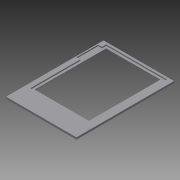
# Autodesk Inventor part: TouchBottom
Saved by Autodesk Inventor 2014 SP1 (Build 180222100, 222)
## iProperties
Created: 2014-03-24
Part Number: TouchBottom
Material: Generic
Document SubType Name: Modeling
Designer: patrigg
Density: 1 g/cm^3
Appearance: Default
Author: patrigg
Autodesk Inventor part; units mm, degrees
ref_plane "YZ Plane" through (0, 0, 0) normal (1, 0, 0) x (0, 1, 0)
ref_plane "XZ Plane" through (0, 0, 0) normal (0, 1, 0) x (-1, 0, 0)
ref_plane "XY Plane" through (0, 0, 0) normal (0, 0, 1) x (1, 0, 0)
sketch "Sketch1" plane through (0, 0, 0) normal (0, 1, 0) x (-1, 0, 0)
  line L0 (-32.5, -45) -> (32.5, -45)
  line L1 (32.5, -45) -> (32.5, 45)
  line L2 (32.5, 45) -> (-32.5, 45)
  line L3 (-32.5, 45) -> (-32.5, -45)
  line L4 (-32.5, -45) -> (32.5, 45) construction
  line L5 (32.5, -45) -> (-32.5, 45) construction
  point P0 (0, 0)
  dimension "d0" = 65
  dimension "d1" = 90
  constraints: 12 end point, 2 midpoint, 2 parallel, 1 horizontal, 1 perpendicular
  measures "d0" distance of L2.end L1.end
  measures "d1" distance of L1.end L0.end
extrude "Extrusion1" add sketch "Sketch1" along normal blind 1.8
sketch "Sketch2" plane through (0, 1.8, 0) normal (0, 1, 0) x (1, 0, 0)
  line L0 (32.5, 45) -> (-32.5, 45) projected
  line L1 (-28, -27) -> (28, -27)
  line L2 (28, -27) -> (28, 43)
  line L3 (28, 43) -> (-28, 43)
  line L4 (-28, 43) -> (-28, -27)
  line L5 (-28, -27) -> (28, 43) construction
  line L6 (28, -27) -> (-28, 43) construction
  line L7 (32.5, -45) -> (32.5, 45) projected
  point P0 (0, 0)
  point P1 (0, 8)
  point P2 (0, 8)
  dimension "d5" = 56
  dimension "d6" = 70
  dimension "d7" = 2
  dimension "d33" = 4.5
  constraints: 12 end point, 3 midpoint, 2 parallel, 1 horizontal, 1 perpendicular
  measures "d5" distance of L3.end L2.end
  measures "d6" distance of L2.end L1.end
  measures "d7" distance between parallel lines of L0 L3
  measures "d33" distance between parallel lines of L7 L2
extrude "Extrusion2" cut sketch "Sketch2" against normal blind 1.1
sketch "Sketch3" plane through (0, 0.7, 0) normal (0, 1, 0) x (1, 0, 0)
  line L0 (28, -27) -> (-28, -27) projected
  line L1 (28, 43) -> (28, -27) projected
  line L2 (-28, 43) -> (28, 43) projected
  line L3 (-28, -27) -> (-28, 43) projected
  line L4 (-26, 41) -> (24, 41)
  line L5 (24, 41) -> (24, -25)
  line L6 (24, -25) -> (-26, -25)
  line L7 (-26, -25) -> (-26, 41)
  point P0 (0, 0)
  dimension "d10" = 2
  dimension "d11" = 2
  dimension "d12" = 4
  dimension "d13" = 2
  constraints: 8 end point, 2 parallel, 1 horizontal, 1 perpendicular
  measures "d10" distance between parallel lines of L2 L4
  measures "d11" distance between parallel lines of L3 L7
  measures "d12" distance between parallel lines of L1 L5
  measures "d13" distance between parallel lines of L0 L6
extrude "Extrusion3" cut sketch "Sketch3" against normal blind 1 contours L4 L5 L6 L7
sketch "Sketch7" plane through (0, 1.8, 0) normal (0, 1, 0) x (1, 0, 0)
  line L0 (-28, -27) -> (-28, 43) projected
  line L1 (32.5, 45) -> (-32.5, 45) projected
  line L2 (-32.5, 45) -> (-32.5, -45) projected
  line L3 (-28, 39) -> (-31.5, 39)
  line L4 (-31.5, 39) -> (-31.5, 19)
  line L5 (-31.5, 19) -> (-28, 19)
  line L6 (-28, 19) -> (-28, 39)
  point P0 (0, 0)
  dimension "d28" = 1
  dimension "d29" = 6
  dimension "d30" = 20
  constraints: 8 end point, 2 parallel, 1 horizontal, 1 perpendicular, 1 point on line
  measures "d28" distance between parallel lines of L4 L2
  measures "d29" distance between parallel lines of L3 L1
  measures "d30" distance between parallel lines of L5 L3
extrude "Extrusion6" cut sketch "Sketch7" against normal up to surface (1.1 mm away)
body "Solid1"
